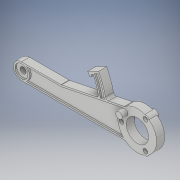
# Autodesk Inventor part: Shock_Arm
Saved by Autodesk Inventor 2019 (Build 230136000, 136)
## iProperties
Created: 2019-03-02
Part Number: Shock_Arm
Material: Generic
Document SubType Name: Modeling
Designer: alarr
Density: 1 g/cm^3
Appearance: Default
Author: alarr
Autodesk Inventor part; units mm, degrees
ref_plane "YZ Plane" through (0, 0, 0) normal (1, 0, 0) x (0, 1, 0)
ref_plane "XZ Plane" through (0, 0, 0) normal (0, 1, 0) x (-1, 0, 0)
ref_plane "XY Plane" through (0, 0, 0) normal (0, 0, 1) x (1, 0, 0)
sketch "Sketch1" plane through (0, 0, 0) normal (0, 0, 1) x (1, 0, 0)
  arc A0 (-15.507236, -18.288) -> (-15.507236, 18.288) centre (0, 0) ccw
  arc A1 (-145.047236, 2.032) -> (-145.047236, -18.288) centre (-145.047236, -8.128) ccw
  line L0 (-15.507236, -18.288) -> (-145.047236, -18.288)
  line L1 (-145.047236, 2.032) -> (-95.224159, 2.032)
  line L2 (-95.224159, 2.032) -> (-15.507236, 18.288)
  arc A2 (-145.047236, -18.288) -> (-145.047236, 2.032) centre (-145.047236, -8.128) ccw construction
  arc A3 (-15.507236, 18.288) -> (-15.507236, -18.288) centre (0, 0) ccw construction
  line L3 (-145.047236, -8.128) -> (-155.207236, -8.128) construction
  line L4 (0, 0) -> (-23.9776, 0) construction
  line L5 (-15.507236, 18.288) -> (-15.507236, 0) construction
  line L6 (-15.507236, -18.288) -> (-15.507236, 0) construction
  line L7 (-145.047236, -8.128) -> (-95.224159, 2.032) construction
  dimension "d0" = 47.9552
  dimension "d1" = 20.32
  dimension "d4" = 139.7
  dimension "d5" = 36.576
  constraints: 16 end point, 10 point on circle, 4 centre point, 2 horizontal, 2 tangent, 1 coincident, 1 collinear, 1 parallel, 1 perpendicular, 1 point on line, 1 vertical
  measures "d0" diameter of A0
  measures "d1" diameter of A1
  measures "d4" horizontal distance of L0.start L3.end
  measures "d5" distance of L2.end L0.start
extrude "Extrusion1" add sketch "Sketch1" along normal blind 10.033
sketch "Sketch2" plane through (0, 0, 10.033) normal (0, 0, 1) x (1, 0, 0)
  arc A0 (-15.507236, -18.288) -> (-15.507236, 18.288) centre (0, 0) ccw
  arc A1 (-145.047236, 2.032) -> (-145.047236, -18.288) centre (-145.047236, -8.128) ccw
  circle A2 centre (-145.047236, -8.128) radius 3.81
  circle A3 centre (0, 0) radius 13.97
  dimension "d8" = 7.62
  dimension "d9" = 27.94
  constraints: 2 centre point, 2 coincident
  measures "d8" diameter of A2
  measures "d9" diameter of A3
extrude "Extrusion2" cut sketch "Sketch2" against normal through all
sketch "Sketch3" plane through (0, 0, 10.033) normal (0, 0, 1) x (1, 0, 0)
  line L0 (0, 0) -> (-19.9644, 0)
  line L1 (0, 0) -> (23.9776, 0) construction
  arc A0 (-15.507236, -18.288) -> (-15.507236, 18.288) centre (0, 0) ccw
  dimension "d61" = 19.9644
  constraints: 4 end point, 2 horizontal, 1 point on circle
  measures "d61" distance of L0.start L0.end
hole "Hole1" at (-19.9644, 0, 10.033) direction (0, 0, -1) diameter 3.175 end through all counterbore diameter 5.715 counterbore depth 3.175
pattern_circular "Circular Pattern1" count 3 over 360 about axis through (0, 0, 10.033) along (0, 0, -1) of "Hole1"
sketch "Sketch5" plane through (0, 0, 10.033) normal (0, 0, 1) x (1, 0, 0)
  circle A0 centre (-145.047236, -8.128) radius 3.81
  arc A1 (-39.274072, 13.44143) -> (-48.460784, 40.082578) centre (-145.047236, -8.128) ccw
  line L0 (-15.507236, 18.288) -> (-95.224159, 2.032) construction
  line L1 (-145.047236, -8.128) -> (-48.460784, 40.082578) construction
  arc A2 (-48.233681, 11.614372) -> (-55.269921, 33.135293) centre (-145.047236, -8.128) ccw
  line L2 (-95.224159, 2.032) -> (-39.274072, 13.44143) construction
  arc A3 (-56.642225, 35.998859) -> (-48.233681, 11.614372) centre (-145.047236, -8.128) ccw construction
  arc A4 (-48.460784, 40.082578) -> (-39.274072, 13.44143) centre (-145.047236, -8.128) ccw construction
  line L3 (-48.460784, 40.082578) -> (-62.096518, 33.276379)
  line L4 (-62.096518, 33.276379) -> (-59.827785, 28.731134)
  line L5 (-59.827785, 28.731134) -> (-57.21427, 30.035656)
  line L6 (-57.21427, 30.035656) -> (-58.065044, 31.740123)
  line L7 (-58.065044, 31.740123) -> (-55.269921, 33.135293)
  arc A5 (-55.269921, 33.135293) -> (-56.642225, 35.998859) centre (-145.047236, -8.128) ccw construction
  line L8 (-48.233681, 11.614372) -> (-39.274072, 13.44143)
  point P0 (0, 0)
  dimension "d29" = 215.9
  dimension "d30" = 9.144
  dimension "d32" = 15
  dimension "d33" = 5.08
  dimension "d34" = 2.921
  dimension "d35" = 3.175
  dimension "d36" = 15.24
  constraints: 16 end point, 10 point on circle, 5 centre point, 4 perpendicular, 4 point on line, 1 coincident, 1 collinear
  measures "d29" diameter of A1
  measures "d30" radial gap between concentric circles of A1 A2
  measures "d32" angle of L0 L1
  measures "d33" distance between parallel lines of L1 L5
  measures "d34" distance between parallel lines of L6 L4
  measures "d35" distance between parallel lines of L3 L7
  measures "d36" distance of L1.end L3.end
extrude "Extrusion4" add sketch "Sketch5" against normal up to surface (10.033 mm away) contours L8 A2 L7 L6 L5 L4 L3 A1
sketch "Sketch4" plane through (0, 0, 10.033) normal (0, 0, 1) x (1, 0, 0)
  circle A0 centre (-145.047236, -8.128) radius 3.81
  arc A1 (-145.047236, 2.032) -> (-145.047236, -18.288) centre (-145.047236, -8.128) ccw
  arc A2 (-138.951236, 0) -> (-138.951236, -16.256) centre (-145.047236, -8.128) ccw construction
  circle A3 centre (-145.047236, -8.128) radius 8.128
  line L0 (-95.224159, 2.032) -> (-145.047236, 2.032)
  line L1 (-145.047236, -18.288) -> (-15.507236, -18.288)
  line L2 (-15.507236, 18.288) -> (-95.224159, 2.032)
  arc A4 (-15.507236, -18.288) -> (-15.507236, 18.288) centre (0, 0) ccw construction
  arc A5 (-17.62577, -16.256) -> (-18.142939, 15.676704) centre (0, 0) ccw construction
  line L3 (-95.019085, 0) -> (-145.047236, 0)
  arc A6 (-145.047236, 0) -> (-145.047236, -16.256) centre (-145.047236, -8.128) ccw
  line L4 (-145.047236, -16.256) -> (-14.742857, -16.256)
  arc A7 (-14.742857, -16.256) -> (-14.578481, 16.403574) centre (0, 0) ccw
  line L5 (-14.578481, 16.403574) -> (-95.019085, 0)
  arc A8 (-138.951236, -16.256) -> (-138.951236, 0) centre (-145.047236, -8.128) ccw
  arc A9 (-18.142939, 15.676704) -> (-17.62577, -16.256) centre (0, 0) ccw
  line L6 (-62.096518, 33.276379) -> (-48.460784, 40.082578)
  arc A10 (-48.233681, 11.614372) -> (-55.269921, 33.135293) centre (-145.047236, -8.128) ccw
  line L7 (-55.269921, 33.135293) -> (-58.065044, 31.740123)
  line L8 (-58.065044, 31.740123) -> (-57.21427, 30.035656)
  line L9 (-57.21427, 30.035656) -> (-59.827785, 28.731134)
  line L10 (-59.827785, 28.731134) -> (-62.096518, 33.276379)
  arc A11 (-39.274072, 13.44143) -> (-48.460784, 40.082578) centre (-145.047236, -8.128) ccw
  arc A12 (-41.265096, 13.035417) -> (-49.38883, 37.348281) centre (-145.047236, -8.128) ccw
  line L11 (-49.38883, 37.348281) -> (-53.934954, 35.07911)
  arc A13 (-46.242657, 12.020385) -> (-53.934954, 35.07911) centre (-145.047236, -8.128) ccw
  line L12 (-46.242657, 12.020385) -> (-41.265096, 13.035417)
  dimension "d24" = 2.032
  dimension "d27" = 2.032
  dimension "d39" = 2.032
  constraints: 16 point on circle, 10 end point, 9 centre point, 4 point on line, 2 coincident, 2 collinear, 2 concentric, 6 other
  measures "d24" radial gap between concentric circles of A2 A3
  measures "d27" distance between parallel lines of L2 L5
  measures "d39" radial gap between concentric circles of A11 A12
extrude "Extrusion3" cut sketch "Sketch4" against normal blind 2.032 contours A3 | L3 L5 A9 L4 A8 | L2 A13 L11 A12
fillet "Fillet1" radius 3.175 4 edges at (-95.2242, 2.032, 5.0165) (-48.2337, 11.6144, 5.0165) (-39.2741, 13.4414, 5.0165) (-15.5072, 18.288, 5.0165)
sketch "Sketch6" plane through (0, 0, 10.033) normal (0, 0, 1) x (1, 0, 0)
  circle A0 centre (-19.9644, 0) radius 2.8575
  circle A1 centre (9.9822, 17.289678) radius 2.8575
  circle A2 centre (9.9822, -17.289678) radius 2.8575
  circle A3 centre (-19.9644, 0) radius 4.8895
  circle A4 centre (0, 0) radius 13.97
  circle A5 centre (9.9822, -17.289678) radius 4.8895
  circle A6 centre (9.9822, 17.289678) radius 4.8895
  dimension "d41" = 9.779
  dimension "d44" = 360
  constraints: 3 centre point, 1 coincident, 7 other
  measures "d41" diameter of A3
extrude "Extrusion5" add sketch "Sketch6" against normal blind 11.938 contours A3 | A5 | A6
sketch "Sketch7" plane through (0, 0, 10.033) normal (0, 0, 1) x (1, 0, 0)
  circle A0 centre (-19.9644, 0) radius 2.8575
  line L0 (-95.019085, 0) -> (-18.142939, 15.676704)
  circle A1 centre (0, 0) radius 19.9644 construction
  circle A2 centre (-15.919865, 12.047206) radius 4.0005
  line L1 (-95.019085, 0) -> (-18.142939, 15.676704)
  dimension "d48" = 8.001
  constraints: 2 centre point, 2 point on circle, 1 coincident, 1 tangent
  measures "d48" diameter of A2
extrude "Extrusion6" add sketch "Sketch7" along normal blind 7.112 contours A2
sketch "Sketch8" plane through (0, 0, 0) normal (0, 0, -1) x (-1, 0, 0)
  circle A0 centre (15.919865, 12.047206) radius 4.0005
  circle A1 centre (15.919865, 12.047206) radius 4.0005
  point P0 (0, 0)
  constraints: 1 centre point, 1 coincident, 1 concentric
extrude "Extrusion7" add sketch "Sketch8" along normal blind 9.652
sketch "Sketch10" plane through (-15.919865, 12.047206, 0) normal (0, 0, -1) x (-1, 0, 0)
  circle A0 centre (0, 0) radius 4.0005 projected
  circle A1 centre (0, 0) radius 4.0005
  circle A2 centre (0, 0) radius 2.032
  point P0 (-15.919865, -12.047206)
  dimension "d58" = 4.064
  constraints: 2 centre point, 2 coincident, 1 concentric
  measures "d58" diameter of A2
extrude "Extrusion9" cut sketch "Sketch10" along normal blind 6.35
full round fillet "Fillet3" first side at (-19.225449, 11.728078, -6.35) centre faces at (-19.86856, 11.40548, -8.551333) second side at (-14.807731, 12.101767, -9.652)
body "Solid1"
